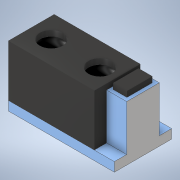
# Autodesk Inventor part: Sharp_Czujnik_Linia
Saved by Autodesk Inventor 2020 (Build 240168000, 168)
## iProperties
Created: 2019-01-30
Part Number: Sharp_Czujnik_Linia
Material: Ogólny
Document SubType Name: Modeling
Designer: atmat
Density: 1 g/cm^3
Appearance: Domyślna
Author: atmat
Autodesk Inventor part; units mm, degrees
sketch "Szkic1" plane through (0, 0, 0) normal (0, 1, 0) x (-1, 0, 0)
  line L0 (7.5, 5) -> (-7.5, 5)
  line L1 (-7.5, 5) -> (-7.5, -5)
  line L2 (-7.5, -5) -> (7.5, -5)
  line L3 (7.5, -5) -> (7.5, 5)
  point P0 (0, 0)
  dimension "d0" = 10
  dimension "d1" = 15
  dimension "d2" = 5
  dimension "d3" = 7.5
  constraints: 8 end point, 2 parallel, 1 horizontal, 1 perpendicular
  measures "d0" distance of L2.end L0.start
  measures "d1" distance of L1.end L2.end
  measures "d2" distance from line of point (0, 0) L2
  measures "d3" distance from line of point (0, 0) L3
extrude "Wyciągnięcie proste1" add sketch "Szkic1" along normal blind 5
sketch "Szkic2" plane through (0, 5, 0) normal (0, 1, 0) x (1, 0, 0)
  line L0 (-7.5, -5) -> (7.5, -5) projected
  line L1 (7.5, -5) -> (7.5, 5) projected
  line L2 (-7.5, -5) -> (7.5, -5)
  line L3 (7.5, -5) -> (7.5, 3)
  line L4 (7.5, 3) -> (-7.5, 3)
  line L5 (-7.5, 3) -> (-7.5, -5)
  point P0 (0, 0)
  dimension "d6" = 8
  constraints: 8 end point, 2 parallel, 1 horizontal, 1 perpendicular, 1 point on line
  measures "d6" distance between parallel lines of L0 L4
extrude "Wyciągnięcie proste2" add sketch "Szkic2" along normal blind 4
sketch "Szkic3" plane through (0, 9, 0) normal (0, 1, 0) x (1, 0, 0)
  circle A0 centre (-4, -1) radius 2
  line L0 (-7.5, 3) -> (-7.5, -5) projected
  line L1 (7.5, 3) -> (-7.5, 3) projected
  circle A1 centre (4.5, -1) radius 2
  line L2 (7.5, -5) -> (7.5, 3) projected
  point P0 (0, 0)
  dimension "d9" = 4
  dimension "d10" = 3.5
  dimension "d11" = 4
  dimension "d12" = 3
  dimension "d13" = 4
  dimension "d14" = 4
  constraints: 2 centre point
  measures "d9" diameter of A0
  measures "d10" distance from line of L0 A0.centre
  measures "d11" distance from line of L1 A0.centre
  measures "d12" distance from line of L2 A1.centre
  measures "d13" distance from line of L1 A1.centre
  measures "d14" diameter of A1
extrude "Wyciągnięcie proste3" cut sketch "Szkic3" against normal blind 1
sketch "Sketch4" plane through (0, 0, 0) normal (0, -1, 0) x (1, 0, 0)
  line L0 (-7.5, 5) -> (7.5, 5) projected
  line L1 (7.5, -5) -> (-7.5, -5) projected
  line L2 (7.5, 5) -> (-7.5, 5)
  line L3 (-7.5, 5) -> (-7.5, -5)
  line L4 (-7.5, -5) -> (7.5, -5)
  line L5 (7.5, 5) -> (11, 5)
  line L6 (11, 5) -> (11, -5)
  line L7 (11, -5) -> (7.5, -5)
  line L8 (7.5, -5) -> (-7.5, -5) projected
  line L9 (-7.5, -5) -> (-7.5, 5) projected
  point P0 (0, 0)
  dimension "d19" = 18.5
  constraints: 12 end point, 2 collinear, 2 parallel, 2 perpendicular, 1 horizontal
  measures "d19" distance between parallel lines of L3 L6
extrude "Extrusion4" add sketch "Sketch4" along normal blind 1.6 separate body
sketch "Sketch5" plane through (0, 0, 0) normal (0, 1, 0) x (1, 0, 0)
  line L0 (11, 2.85) -> (7.5, 2.85)
  line L1 (7.5, 2.85) -> (7.5, -2.85)
  line L2 (7.5, -2.85) -> (11, -2.85)
  line L3 (11, -2.85) -> (11, 2.85)
  line L4 (-7.5, 5) -> (11, 5) projected
  line L5 (7.5, -5) -> (7.5, 3) projected
  point P0 (0, 0)
  dimension "d20" = 3.5
  dimension "d21" = 5.7
  dimension "d22" = 2.15
  dimension "d23" = 0
  constraints: 8 end point, 2 parallel, 1 horizontal, 1 perpendicular
  measures "d20" distance of L1.end L2.end
  measures "d21" distance of L2.end L0.start
  measures "d22" distance between parallel lines of L4 L0
  measures "d23" distance between parallel lines of L5 L1
extrude "Extrusion5" add sketch "Sketch5" along normal blind 8 bodies 2
sketch "Sketch7" plane through (0, 8, 0) normal (0, 1, 0) x (1, 0, 0)
  line L0 (10.4, 2.2) -> (8, 2.2)
  line L1 (8, 2.2) -> (8, -2.2)
  line L2 (8, -2.2) -> (10.4, -2.2)
  line L3 (10.4, -2.2) -> (10.4, 2.2)
  line L4 (7.5, -2.85) -> (11, -2.85) projected
  line L5 (7.5, 2.85) -> (7.5, -2.85) projected
  point P0 (0, 0)
  dimension "d32" = 4.4
  dimension "d33" = 0.65
  dimension "d34" = 2.4
  dimension "d35" = 0.5
  constraints: 8 end point, 2 parallel, 1 horizontal, 1 perpendicular
  measures "d32" distance of L2.end L0.start
  measures "d33" distance between parallel lines of L4 L2
  measures "d34" distance of L1.end L2.end
  measures "d35" distance between parallel lines of L5 L1
extrude "Extrusion7" add sketch "Sketch7" along normal blind 1 bodies 2
ref_plane "Work Plane1" through (-7.5, 0, 3) normal (0, 0, 1) x (1, 0, 0)
ref_plane "Work Plane2" through (8, 8, 1.2) normal (0, 0, 1) x (1, 0, 0)
ref_plane "Work Plane3" through (10.4, 8, -1.2) normal (0, 0, -1) x (-1, 0, 0)
ref_plane "Work Plane4" through (-7.5, 0, 0) normal (0, 0, 1) x (1, 0, 0)
sketch "Sketch9" plane through (8, 8, 1.2) normal (0, 0, 1) x (1, 0, 0)
  line L0 (1.4, 1) -> (2.3459, 4)
  line L1 (2.3459, 4) -> (0.0541, 4)
  line L2 (0.0541, 4) -> (1, 1)
  line L3 (1, 1) -> (1.4, 1)
  line L4 (0, 1) -> (2.4, 1) projected
  line L5 (2.4, 0) -> (2.4, 1) projected
  line L6 (2.4, 1) -> (0, 1) construction
  line L7 (1.2, 1) -> (1.2, 8.0865) construction
  line L8 (-15.5, 1) -> (-0.5, 1) construction
  line L9 (1.2, 1) -> (1.2, 4)
  point P0 (-8, -8)
  dimension "d47" = 0.4
  dimension "d48" = 0
  dimension "d49" = 1
  dimension "d50" = 17.5
  dimension "d51" = 35
  dimension "d53" = 3
  constraints: 12 end point, 2 midpoint, 1 horizontal, 1 parallel, 1 vertical
  measures "d47" distance of L2.end L0.start
  measures "d48" distance between parallel lines of L4 L3
  measures "d49" distance from line of L5 L0.start
  measures "d50" angle of L0 L7
  measures "d51" angle of L0 L2
  measures "d53" distance between parallel lines of L8 L1
body "Solid2"
